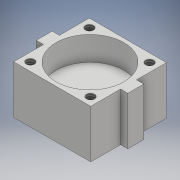
# Autodesk Inventor part: teflonlense assem
Saved by Autodesk Inventor 2018 (Build 220112000, 112)
## iProperties
Created: 2018-10-24
Part Number: teflonlense assem
Material: Generic
Document SubType Name: Modeling
Designer: STS
Density: 1 g/cm^3
Appearance: Default
Author: STS
Autodesk Inventor part; units mm, degrees
ref_plane "YZ Plane" through (0, 0, 0) normal (1, 0, 0) x (0, 1, 0)
ref_plane "XZ Plane" through (0, 0, 0) normal (0, 1, 0) x (-1, 0, 0)
ref_plane "XY Plane" through (0, 0, 0) normal (0, 0, 1) x (1, 0, 0)
sketch "Sketch1" plane through (0, 0, 0) normal (0, 0, 1) x (1, 0, 0)
  line L0 (8, -7.85) -> (-8, -7.85)
  line L1 (-8, 7.85) -> (8, 7.85)
  line L2 (8, -7.85) -> (-8, 7.85) construction
  line L3 (-9.5, -1.65) -> (-9.5, 1.65)
  line L4 (9.5, 1.65) -> (9.5, -1.65)
  line L5 (-8, -7.85) -> (-8, -1.65)
  line L6 (-8, 1.65) -> (-8, 7.85)
  line L7 (8, 7.85) -> (8, 1.65)
  line L8 (8, -1.65) -> (8, -7.85)
  line L9 (9.5, -1.65) -> (8, -1.65)
  line L10 (-8, -1.65) -> (-9.5, -1.65)
  line L11 (-9.5, 1.65) -> (-8, 1.65)
  line L12 (8, 1.65) -> (9.5, 1.65)
  point P0 (0, 0)
  dimension "d0" = 16
  dimension "d1" = 15.7
  dimension "d2" = 19
  dimension "d3" = 3.3
  constraints: 26 end point, 10 parallel, 4 perpendicular, 3 horizontal, 1 midpoint
  measures "d0" distance of L1.start L1.end
  measures "d1" distance of L0.end L1.start
  measures "d2" distance of L3.end L4.start
  measures "d3" distance of L3.start L3.end
extrude "Extrusion1" add sketch "Sketch1" along normal blind 10
sketch "Sketch2" plane through (0, 0, 10) normal (0, 0, 1) x (1, 0, 0)
  circle A0 centre (0, 0) radius 7.05
  dimension "d6" = 14.1
  constraints: 1 centre point, 1 coincident
  measures "d6" diameter of A0
extrude "Extrusion2" cut sketch "Sketch2" against normal blind 5
sketch "Sketch4" plane through (0, 0, 10) normal (0, 0, 1) x (1, 0, 0)
  circle A0 centre (0, 0) radius 8.75
  line L0 (-8, 1.65) -> (-8, 7.85) projected
  line L1 (0, 0) -> (-8, 7.85)
  line L2 (-8, -1.65) -> (-8, -7.85) projected
  line L3 (0, 0) -> (-8, -7.85)
  line L4 (-8, -7.85) -> (8, -7.85) projected
  line L5 (0, 0) -> (8, -7.85)
  line L6 (8, 7.85) -> (-8, 7.85) projected
  line L7 (0, 0) -> (8, 7.85)
  point P0 (-6.2455, 6.1284)
  point P1 (6.2455, 6.1284)
  point P2 (6.2455, -6.1284)
  point P3 (-6.2455, -6.1284)
  dimension "d17" = 17.5
  constraints: 8 end point, 4 point on circle, 4 point on line, 2 collinear, 1 centre point, 1 coincident
  measures "d17" diameter of A0
hole "Hole2" at (-6.2455, 6.1284, 10) at (6.2455, 6.1284, 10) at (6.2455, -6.1284, 10) at (-6.2455, -6.1284, 10) direction (0, 0, -1) diameter 1.694 end through all thread size "2-56 UNC" class "2B" standard "ANSI Unified Screw Threads"
body "Solid1"
